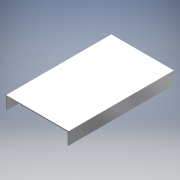
# Autodesk Inventor part: Mottor Protection Piece
Saved by Autodesk Inventor 2019 (Build 230136000, 136)
## iProperties
Created: 2019-11-02
Part Number: Mottor Protection Piece
Material: Aluminum 6061
Document SubType Name: Modeling
Designer: admin
Density: 2.7 g/cm^3
Appearance: Aluminum - Flat
Author: admin
Autodesk Inventor part; units mm, degrees
ref_plane "YZ Plane" through (0, 0, 0) normal (1, 0, 0) x (0, 1, 0)
ref_plane "XZ Plane" through (0, 0, 0) normal (0, 1, 0) x (-1, 0, 0)
ref_plane "XY Plane" through (0, 0, 0) normal (0, 0, 1) x (1, 0, 0)
sketch "Sketch1" plane through (0, 0, 0) normal (0, 0, 1) x (1, 0, 0)
  line L0 (0, 0) -> (0, 25)
  line L1 (0, 25) -> (125, 25)
  line L2 (125, 25) -> (125, 0)
  line L3 (123, 0) -> (123, 23)
  line L4 (123, 23) -> (2, 23)
  line L5 (2, 23) -> (2, 0)
  line L6 (0, 0) -> (2, 0)
  line L7 (123, 0) -> (125, 0)
  dimension "d0" = 25
  dimension "d1" = 125
  dimension "d2" = 25
  dimension "d3" = 2
  constraints: 16 end point, 4 perpendicular, 1 collinear, 1 horizontal, 1 vertical, 2 other
  measures "d0" distance of L0.start L0.end
  measures "d1" distance of L0.end L1.end
  measures "d2" distance of L1.end L2.end
  measures "d3" distance between parallel lines of L1 L4
extrude "Extrusion1" add sketch "Sketch1" along normal mid plane 210
sketch "Sketch2" plane through (125, 0, 105) normal (1, 0, 0) x (0, 0, -1)
  line L0 (-37.1075, -32.7019) -> (-16.9826, -51.5645) projected
  arc A0 (-19.3607, -56.7355) -> (-16.9826, -51.5645) centre (-19.0342, -53.7534) ccw projected
  line L1 (-19.3607, -56.7355) -> (-50.4892, -53.3266) projected
  arc A1 (-50.4892, -53.3266) -> (-55.5556, -43.1569) centre (-69.9997, -56.6998) ccw projected
  line L2 (-55.5556, -43.1569) -> (-48.2423, -32.0821) projected
  arc A2 (-48.2423, -32.0821) -> (-37.1075, -32.7019) centre (-41.913, -18.7038) ccw projected
  line L3 (-75.1262, -21.5392) -> (-58.7293, -21.5392) projected
  arc A3 (-55.8951, -23.5557) -> (-58.7293, -21.5392) centre (-58.7293, -24.5392) ccw projected
  arc A4 (-55.8951, -23.5557) -> (-54.2437, -26.8888) centre (-41.913, -18.7038) ccw projected
  arc A5 (-54.3157, -30.3107) -> (-54.2437, -26.8888) centre (-56.7431, -28.5479) ccw projected
  line L4 (-54.3157, -30.3107) -> (-59.3237, -37.207) projected
  arc A6 (-62.8365, -38.2409) -> (-59.3237, -37.207) centre (-61.7512, -35.4442) ccw projected
  arc A7 (-62.8365, -38.2409) -> (-89.7654, -57.8643) centre (-69.9997, -56.6998) ccw projected
  arc A8 (-91.9651, -60.9335) -> (-89.7654, -57.8643) centre (-92.7603, -58.0408) ccw projected
  arc A9 (-94.9604, -58.1017) -> (-91.9651, -60.9335) centre (-91.9651, -57.9335) ccw projected
  arc A10 (-90.8616, -42.9236) -> (-94.9604, -58.1017) centre (-69.9997, -56.6998) ccw projected
  line L5 (-90.8616, -42.9236) -> (-77.6297, -22.886) projected
  arc A11 (-75.1262, -21.5392) -> (-77.6297, -22.886) centre (-75.1262, -24.5392) ccw projected
  line L6 (14.2601, -42.0875) -> (14.5644, -34.6181) projected
  arc A12 (16.26, -32.0374) -> (14.5644, -34.6181) centre (17.5619, -34.7402) ccw projected
  arc A13 (16.26, -32.0374) -> (22.9996, -25.4705) centre (9.837, -18.7038) ccw projected
  arc A14 (25.6676, -23.8421) -> (22.9996, -25.4705) centre (25.6676, -26.8421) ccw projected
  line L7 (25.6676, -23.8421) -> (32.9459, -23.8421) projected
  arc A15 (35.7755, -27.8386) -> (32.9459, -23.8421) centre (32.9459, -26.8421) ccw projected
  arc A16 (20.9479, -43.8593) -> (35.7755, -27.8386) centre (9.837, -18.7038) ccw projected
  line L8 (20.9479, -43.8593) -> (18.4697, -44.9538) projected
  arc A17 (14.2601, -42.0875) -> (18.4697, -44.9538) centre (17.2576, -42.2096) ccw projected
  arc A18 (-57.5249, -72.0757) -> (-51.5712, -63.9406) centre (-69.9997, -56.6998) ccw projected
  arc A19 (-48.3568, -62.0675) -> (-51.5712, -63.9406) centre (-48.779, -65.0377) ccw projected
  line L9 (-48.3568, -62.0675) -> (-37.4982, -63.611) projected
  arc A20 (-36.7083, -69.3254) -> (-37.4982, -63.611) centre (-37.9204, -66.5811) ccw projected
  line L10 (-36.7083, -69.3254) -> (-54.4227, -77.1496) projected
  arc A21 (-57.5249, -72.0757) -> (-54.4227, -77.1496) centre (-55.6348, -74.4054) ccw projected
  line L11 (-76.583, -76.7389) -> (-76.583, -78.0382) projected
  arc A22 (-79.3294, -79.8937) -> (-76.583, -78.0382) centre (-78.583, -78.0382) ccw projected
  arc A23 (-88.2867, -73.7464) -> (-79.3294, -79.8937) centre (-69.9997, -56.6998) ccw projected
  arc A24 (-86.8237, -70.3827) -> (-88.2867, -73.7464) centre (-86.8237, -72.3827) ccw projected
  line L12 (-86.8237, -70.3827) -> (-85.142, -70.3827) projected
  arc A25 (-83.7528, -70.9439) -> (-85.142, -70.3827) centre (-85.142, -72.3827) ccw projected
  arc A26 (-83.7528, -70.9439) -> (-77.7955, -74.9005) centre (-69.9997, -56.6998) ccw projected
  arc A27 (-76.583, -76.7389) -> (-77.7955, -74.9005) centre (-78.583, -76.7389) ccw projected
  line L13 (14.6425, -2.7064) -> (14.6425, 4.5196) projected
  arc A28 (18.5982, 7.3633) -> (14.6425, 4.5196) centre (17.6425, 4.5196) ccw projected
  arc A29 (35.7755, -9.5689) -> (18.5982, 7.3633) centre (9.837, -18.7038) ccw projected
  arc A30 (32.9459, -13.5655) -> (35.7755, -9.5689) centre (32.9459, -10.5655) ccw projected
  line L14 (32.9459, -13.5655) -> (25.6676, -13.5655) projected
  arc A31 (22.9996, -11.9371) -> (25.6676, -13.5655) centre (25.6676, -10.5655) ccw projected
  arc A32 (22.9996, -11.9371) -> (16.3269, -5.4026) centre (9.837, -18.7038) ccw projected
  arc A33 (14.6425, -2.7064) -> (16.3269, -5.4026) centre (17.6425, -2.7064) ccw projected
  line L15 (-41.913, 8.7962) -> (-41.4503, 8.7962) projected
  arc A34 (-38.6444, 4.7345) -> (-41.4503, 8.7962) centre (-41.4503, 5.7962) ccw projected
  line L16 (-38.6444, 4.7345) -> (-41.2275, -2.0922) projected
  arc A35 (-43.676, -4.0092) -> (-41.2275, -2.0922) centre (-44.0334, -1.0305) ccw projected
  arc A36 (-43.676, -4.0092) -> (-55.8951, -13.8519) centre (-41.913, -18.7038) ccw projected
  arc A37 (-58.7293, -15.8684) -> (-55.8951, -13.8519) centre (-58.7293, -12.8684) ccw projected
  line L17 (-58.7293, -15.8684) -> (-67.4194, -15.8684) projected
  arc A38 (-69.9228, -11.2152) -> (-67.4194, -15.8684) centre (-67.4194, -12.8684) ccw projected
  line L18 (-69.9228, -11.2152) -> (-64.861, -3.5499) projected
  arc A39 (-41.913, 8.7962) -> (-64.861, -3.5499) centre (-41.913, -18.7038) ccw projected
  line L19 (-27.6338, -22.5955) -> (-4.4421, -22.5955) projected
  arc A40 (-4.4421, -22.5955) -> (3.4115, -32.0362) centre (9.837, -18.7038) ccw projected
  arc A41 (5.0262, -35.4387) -> (3.4115, -32.0362) centre (2.109, -34.7387) ccw projected
  line L20 (5.0262, -35.4387) -> (1.9259, -48.3584) projected
  arc A42 (-2.7541, -50.0859) -> (1.9259, -48.3584) centre (-0.9913, -47.6584) ccw projected
  line L21 (-2.7541, -50.0859) -> (-31.494, -29.215) projected
  arc A43 (-31.494, -29.215) -> (-27.6338, -22.5955) centre (-41.913, -18.7038) ccw projected
  line L22 (-6.5747, -14.8121) -> (-25.5012, -14.8121) projected
  arc A44 (-28.2673, -12.9736) -> (-25.5012, -14.8121) centre (-25.5012, -11.8121) ccw projected
  arc A45 (-28.2673, -12.9736) -> (-34.4604, -5.9171) centre (-41.913, -18.7038) ccw projected
  arc A46 (-35.5882, -1.8976) -> (-34.4604, -5.9171) centre (-32.9497, -3.3252) ccw projected
  line L23 (-35.5882, -1.8976) -> (-30.653, 7.2238) projected
  arc A47 (-28.0144, 8.7962) -> (-30.653, 7.2238) centre (-28.0144, 5.7962) ccw projected
  line L24 (-28.0144, 8.7962) -> (-0.4202, 8.7962) projected
  arc A48 (2.5798, 5.7962) -> (-0.4202, 8.7962) centre (-0.4202, 5.7962) ccw projected
  line L25 (2.5798, 5.7962) -> (2.5798, -4.1563) projected
  arc A49 (1.3085, -6.6081) -> (2.5798, -4.1563) centre (-0.4202, -4.1563) ccw projected
  arc A50 (1.3085, -6.6081) -> (-3.8087, -12.9736) centre (9.837, -18.7038) ccw projected
  arc A51 (-6.5747, -14.8121) -> (-3.8087, -12.9736) centre (-6.5747, -11.8121) ccw projected
  circle A52 centre (-81.913, -5.781) radius 2.75 projected
  circle A53 centre (7.837, -58.4172) radius 2.75 projected
  circle A54 centre (-19.913, 17.776) radius 2.75 projected
  circle A55 centre (-109.9997, -47.6996) radius 2.75 projected
  circle A56 centre (43.4223, 4.8129) radius 2.75 projected
  line L26 (-25.906, 18.0659) -> (-40.1014, 18.7524) projected
  arc A57 (-40.1014, 18.7524) -> (-73.2057, 1.9606) centre (-41.913, -18.7038) ccw projected
  line L27 (-73.2057, 1.9606) -> (-76.5462, -3.0981) projected
  arc A58 (-76.5462, -3.0981) -> (-82.2729, -11.7702) centre (-81.913, -5.781) ccw projected
  line L28 (-82.2729, -11.7702) -> (-99.2063, -37.4131) projected
  arc A59 (-99.2063, -37.4131) -> (-101.6224, -41.6996) centre (-69.9997, -56.6998) ccw projected
  line L29 (-101.6224, -41.6996) -> (-109.9997, -41.6996) projected
  arc A60 (-109.9997, -41.6996) -> (-109.9997, -53.6996) centre (-109.9997, -47.6996) ccw projected
  line L30 (-109.9997, -53.6996) -> (-104.8709, -53.6996) projected
  arc A61 (-104.8709, -53.6996) -> (-54.959, -88.3032) centre (-69.9997, -56.6998) ccw projected
  line L31 (-54.959, -88.3032) -> (2.4193, -60.9957) projected
  arc A62 (2.4193, -60.9957) -> (13.2548, -55.8388) centre (7.837, -58.4172) ccw projected
  line L32 (13.2548, -55.8388) -> (24.8778, -50.3072) projected
  arc A63 (24.8778, -50.3072) -> (42.845, -7.0644) centre (9.837, -18.7038) ccw projected
  line L33 (42.845, -7.0644) -> (48.4494, 1.5375) projected
  arc A64 (48.4494, 1.5375) -> (42.0639, 10.6571) centre (43.4223, 4.8129) ccw projected
  line L34 (42.0639, 10.6571) -> (32.0639, 8.3327) projected
  arc A65 (32.0639, 8.3327) -> (11.5279, 16.2554) centre (9.837, -18.7038) ccw projected
  line L35 (11.5279, 16.2554) -> (-13.92, 17.4862) projected
  arc A66 (-13.92, 17.4862) -> (-25.906, 18.0659) centre (-19.913, 17.776) ccw projected
  circle A67 centre (-69.9997, -56.6998) radius 9.8 projected
  circle A68 centre (-41.913, -18.7038) radius 9.8 projected
  circle A69 centre (9.837, -18.7038) radius 9.8 projected
  circle A70 centre (35, 17) radius 2.75
  circle A71 centre (105, 12.5) radius 2.75
  line L36 (105, 0) -> (105, 25)
  line L37 (0, 25) -> (210, 25) projected
  line L38 (0, 0) -> (0, 25) projected
  circle A72 centre (166.5777, 4.8129) radius 2.75
  circle A73 centre (175, 17) radius 2.75
  circle A74 centre (105, 12.5) radius 2.75
  dimension "d6" = 5.5
  dimension "d7" = 5.5
  dimension "d8" = 8
  dimension "d9" = 12.5
  dimension "d10" = 35
  constraints: 5 centre point, 2 end point, 2 midpoint, 2 symmetric about line, 3 other
  measures "d6" diameter of A70
  measures "d7" diameter of A71
  measures "d8" distance from line of L37 A70.centre
  measures "d9" distance from line of L37 A71.centre
  measures "d10" distance from line of L38 A70.centre
extrude "Extrusion2" cut sketch "Sketch2" against normal blind 205.75 contours A56 | A70 | A71 L36 | L36 A71 | A72 | A73
body "Solid1"
